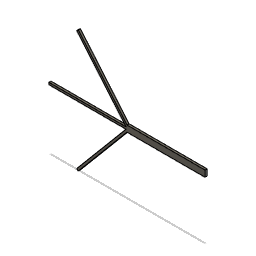
cross_junction (Autodesk Fusion 360 design; units mm, degrees)
Autodesk Fusion 360 part; units mm, degrees
note: some values were not read from the file. Set by a fixed rule: which sketch regions a step uses.
sketch "Sketch1" plane through (0, 0, 0) normal (0, 0, 1) x (1, 0, 0)
  line L0 (0, 0) -> (25, 0) construction
  line L1 (2.8272, -5.8688) -> (7.5, -0.3)
  line L2 (7.5, 0.3) -> (15, 0.3)
  line L3 (15, 0.3) -> (15, -0.3)
  line L4 (15, -0.3) -> (7.5, -0.3)
  line L5 (7.5, -0.3) -> (7.5, 0.3)
  line L6 (0, 0.1) -> (7.5, 0.1)
  line L7 (7.5, 0.1) -> (7.5, -0.1)
  line L8 (7.5, -0.1) -> (0, -0.1)
  line L9 (0, -0.1) -> (0, 0.1)
  circle A0 centre (7.5, 0) radius 7.5 construction
  line L10 (7.4067, -0.1) -> (2.674, -5.7403)
  line L11 (2.8272, -5.8688) -> (2.674, -5.7403)
  line L12 (2.8272, 5.8688) -> (7.5, 0.3)
  line L13 (7.4067, 0.1) -> (2.674, 5.7403)
  line L14 (2.8272, 5.8688) -> (2.674, 5.7403)
  point P0 (2.7506, -5.8046)
  point P1 (7.5, 0)
  point P2 (2.7506, -5.8046)
  point P3 (2.7506, -5.8046)
  point P4 (2.7506, -5.8046)
  dimension "d39" = 25
  dimension "d42" = 0.6
  dimension "d49" = 0.2
  dimension "d50" = 15
  dimension "d51" = 7.5
  dimension "d52" = 0.2
  dimension "d53" = 50
  dimension "d54" = 5.8046
  dimension "d55" = 2.7506
  constraint coincident L0.start origin
  constraint horizontal L2
  constraint vertical L3
  constraint horizontal L4
  constraint vertical L5
  constraint midpoint L5 P1
  constraint horizontal L0
  constraint horizontal L6
  constraint vertical L7
  constraint horizontal L8
  constraint vertical L9
  constraint midpoint L0.start L9
  constraint coincident P1 A0.centre
  constraint coincident L0.start A0
  constraint coincident P4 A0
  constraint coincident L1.end L4.end
  constraint coincident L0 P1
  constraint coincident L7 P1
  constraint coincident L8 L10.start
  constraint parallel L1 L10
  constraint perpendicular L1 L11
  constraint coincident P4 L11
  constraint midpoint P4 L11
  constraint symmetric L0 L1.start L12.start
  constraint symmetric L0 L1.end L2.start
  constraint symmetric L0 L10.start L13.start
  constraint symmetric L0 L10.end L13.end
  constraint coincident P4 P3
  measures "d39" distance of L0.start L0.end
  measures "d42" distance of L2.start L1.end
  measures "d49" distance of L6.start L8.end
  measures "d50" horizontal distance of L3.end L8.end
  measures "d51" distance of L3.end L1.end
  measures "d52" distance of L1 L10
  measures "d53" angle of L0 L10
  measures "d54" distance of P4 L0
  measures "d55" horizontal distance of L0.start P4
extrude "Extrude1" add sketch "Sketch1" along normal blind 0.2
ref_plane "WorkPlane1" through (5.087, -3.0201, 0.1) normal (0.766044, -0.642788, 0) x (0.642788, 0.766044, 0)
equation "d1001 = depth"
equation "channelwidth = 0.2 mm"
equation "depth = 0.2 mm"
equation "length = 15 mm"
equation "d42 = channelwidth * 3"
equation "angle = 50 deg"
equation "d49 = channelwidth"
equation "d50 = length"
equation "d51 = length / 2"
equation "d52 = channelwidth"
equation "d53 = angle"
